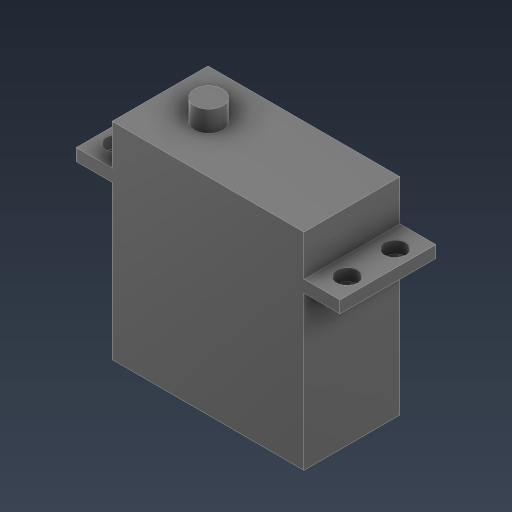
# Autodesk Inventor part: feetech_25kg_servo
Saved by Autodesk Inventor 2024 (Build 280153000, 153)
## iProperties
Created: 2025-07-06
Part Number: feetech_25kg_servo
Material: Acetal Resin, Black
Document SubType Name: Modeling
Designer: Piter
Density: 1.425 g/cm^3
Appearance: Smooth - Black
Author: Piter
Autodesk Inventor part; units mm, degrees
ref_plane "YZ Plane" through (0, 0, 0) normal (1, 0, 0) x (0, 1, 0)
ref_plane "XZ Plane" through (0, 0, 0) normal (0, 1, 0) x (-1, 0, 0)
ref_plane "XY Plane" through (0, 0, 0) normal (0, 0, 1) x (1, 0, 0)
sketch "Sketch1" plane through (0, 0, 0) normal (0, 1, 0) x (-1, 0, 0)
  line L0 (-20, 10) -> (20, 10)
  line L1 (20, 10) -> (20, -10)
  line L2 (20, -10) -> (-20, -10)
  line L3 (-20, -10) -> (-20, 10)
  line L4 (-20, 10) -> (20, -10) construction
  line L5 (20, 10) -> (-20, -10) construction
  point P0 (0, 0)
  dimension "d0" = 40
  dimension "d1" = 20
  constraints: 12 end point, 2 midpoint, 2 parallel, 1 horizontal, 1 perpendicular
  measures "d0" distance of L1.end L2.end
  measures "d1" distance of L0.end L1.end
extrude "Extrusion1" add sketch "Sketch1" along normal blind 43
sketch "Sketch2" plane through (-20, 0, 10) normal (0, 0, 1) x (1, 0, 0)
  line L0 (-7.5, 34.5) -> (47.5, 34.5)
  line L1 (47.5, 34.5) -> (47.5, 32)
  line L2 (47.5, 32) -> (-7.5, 32)
  line L3 (-7.5, 32) -> (-7.5, 34.5)
  line L4 (0, 0) -> (40, 0) projected
  line L5 (0, 0) -> (0, 43) projected
  point P0 (20, 0)
  point P1 (-7.5, 33.25)
  dimension "d4" = 55
  dimension "d5" = 2.5
  dimension "d6" = 32
  dimension "d7" = 7.5
  constraints: 8 end point, 2 parallel, 1 horizontal, 1 midpoint, 1 perpendicular
  measures "d4" distance of L1.end L2.end
  measures "d5" distance of L0.end L1.end
  measures "d6" distance between parallel lines of L4 L2
  measures "d7" distance from line of point (-7.5, 33.25) L5
extrude "Extrusion2" add sketch "Sketch2" against normal up to surface (20 mm away)
sketch "Sketch3" plane through (-27.5, 34.5, 10) normal (0, 1, 0) x (1, 0, 0)
  line L0 (0, 0) -> (0, 20) projected
  line L1 (0, 10) -> (55, 10) construction
  line L2 (55, 0) -> (55, 20) projected
  line L3 (7.5, 0) -> (47.5, 0) projected
  line L4 (27.5, 0) -> (27.5, 20) construction
  line L5 (47.5, 20) -> (7.5, 20) projected
  circle A0 centre (3.5, 5) radius 2.25
  circle A1 centre (3.5, 15) radius 2.25
  circle A2 centre (51.5, 5) radius 2.25
  circle A3 centre (51.5, 15) radius 2.25
  point P0 (27.5, 10)
  dimension "d10" = 4.5
  dimension "d11" = 5
  dimension "d12" = 24
  constraints: 4 centre point, 4 end point, 4 midpoint, 3 symmetric about line, 3 other
  measures "d10" diameter of A0
  measures "d11" distance from line of L1 A0.centre
  measures "d12" distance from line of L4 A0.centre
extrude "Extrusion3" cut sketch "Sketch3" against normal through all
sketch "Sketch4" plane through (0, 43, 0) normal (0, 1, 0) x (1, 0, 0)
  line L0 (-27.5, -10) -> (-27.5, 10) projected
  line L1 (-27.5, 0) -> (27.5, 0) construction
  line L2 (27.5, -10) -> (27.5, 10) projected
  line L3 (0, -10) -> (0, 10) construction
  line L4 (20, 10) -> (-20, 10) projected
  circle A0 centre (-9.86, 0) radius 3
  point P0 (0, 0)
  dimension "d15" = 6
  dimension "d16" = 9.86
  constraints: 4 end point, 3 midpoint, 1 centre point, 1 point on line
  measures "d15" diameter of A0
  measures "d16" distance from line of L3 A0.centre
extrude "Extrusion4" add sketch "Sketch4" along normal blind 4.38
body "Solid1"
